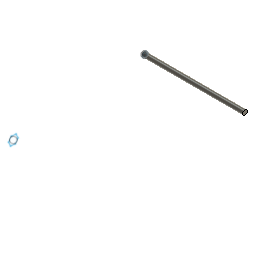
handler (Autodesk Fusion 360 design; units mm, degrees)
part number: 2026-05-17-19-38-54-358
Autodesk Fusion 360 part; units mm, degrees
sketch "handler" plane through (0, 0, 0) normal (1, 0, 0) x (0, 1, 0)
  circle A0 centre (100, 100) radius 2.375
  point P0 (100, 100)
  dimension "d4" = 4.75
  constraint coincident P0 A0.centre
  measures "d4" diameter of A0
extrude "Extrude2" add sketch "handler" along normal blind 100
sketch "main" plane through (0, 0, 0) normal (1, 0, 0) x (0, 1, 0)
  line L0 (-33.7556, 87.8206) -> (-29.079, 87.3528)
  line L1 (-29.079, 87.3528) -> (-26.3355, 91.169)
  line L2 (-26.3355, 91.169) -> (-28.2688, 95.453)
  line L3 (-28.2688, 95.453) -> (-32.9454, 95.9208)
  line L4 (-32.9454, 95.9208) -> (-35.6889, 92.1046)
  line L5 (-35.6889, 92.1046) -> (-33.7556, 87.8206)
  point P0 (-31.0122, 91.6368)
  dimension "d7" = 4.7
  measures "d7" distance of L0.start P0
extrude "Extrude1" [suppressed]
named bodies: "handler"
